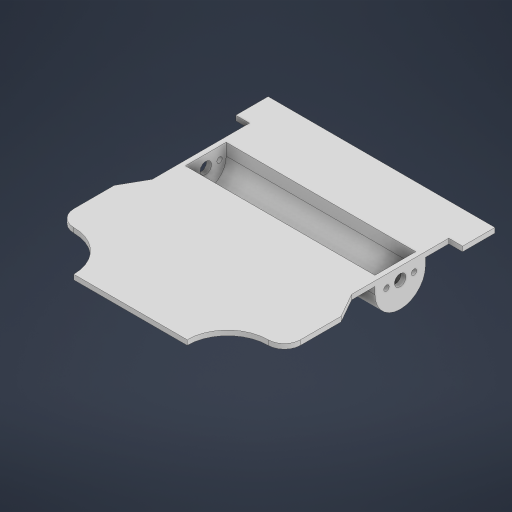
# Autodesk Inventor part: karoserie1
Saved by Autodesk Inventor 2023 (Build 270158000, 158)
## iProperties
Created: 2024-04-14
Part Number: karoserie1
Material: Generic
Document SubType Name: Modeling
Designer: Matooš
Density: 1 g/cm^3
Appearance: Default
Author: Matooš
Autodesk Inventor part; units mm, degrees
ref_plane "YZ Plane" through (0, 0, 0) normal (1, 0, 0) x (0, 1, 0)
ref_plane "XZ Plane" through (0, 0, 0) normal (0, 1, 0) x (-1, 0, 0)
ref_plane "XY Plane" through (0, 0, 0) normal (0, 0, 1) x (1, 0, 0)
sketch "Sketch1" plane through (0, 0, 0) normal (0, 1, 0) x (-1, 0, 0)
  line L0 (70, 45) -> (61.5, 30)
  line L1 (61.5, 30) -> (61.5, -30)
  line L2 (61.5, -30) -> (70, -30)
  line L3 (70, -30) -> (70, -50)
  line L4 (70, -50) -> (-70, -50)
  line L5 (-70, -50) -> (-70, -30)
  line L6 (-70, -30) -> (-61.5, -30)
  line L7 (-61.5, -30) -> (-61.5, 30)
  line L8 (-61.5, 30) -> (-70, 45)
  line L9 (70, 45) -> (70, 80)
  line L10 (-70, 45) -> (-70, 80)
  line L11 (35, 105) -> (-35, 105)
  line L12 (-98, 0) -> (98, 0) projected
  line L13 (0, -81) -> (0, 136) projected
  line L14 (70, 80) -> (35, 80)
  line L15 (35, 80) -> (35, 105)
  line L16 (-35, 105) -> (-35, 80)
  line L17 (-35, 80) -> (-70, 80)
  point P0 (0, 0)
  dimension "d0" = 60
  dimension "d1" = 60
  dimension "d2" = 123
  dimension "d3" = 140
  dimension "d4" = 20
  dimension "d5" = 140
  dimension "d8" = 35
  dimension "d15" = 30
  dimension "d45" = 15
  dimension "d46" = 15
  dimension "d47" = 35
  dimension "d48" = 70
  dimension "d49" = 155
  constraints: 32 end point, 9 perpendicular, 2 horizontal, 2 vertical, 1 collinear, 4 other
  measures "d0" distance of L0.end L1.end
  measures "d1" distance of L6.end L7.end
  measures "d2" distance between parallel lines of L7 L1
  measures "d3" distance of L3.end L4.end
  measures "d4" distance between parallel lines of L4 L2
  measures "d5" distance between parallel lines of L10 L9
  measures "d8" distance of L10.end L8.end
  measures "d15" distance between parallel lines of L12 L6
  measures "d45" vertical distance of L0.start L0.end
  measures "d46" vertical distance of L7.end L8.end
  measures "d47" distance of L0.start L9.end
  measures "d48" distance of L11.start L11.end
  measures "d49" distance between parallel lines of L4 L11
extrude "Extrusion1" add sketch "Sketch1" along normal blind 3
sketch "Sketch2" plane through (0, 0, 0) normal (0, -1, 0) x (1, 0, 0)
  line L0 (-98, 0) -> (98, 0) projected
  line L1 (0, 136) -> (0, -81) projected
  line L2 (61.5, 15.6) -> (58.5, 15.6)
  line L3 (58.5, 15.6) -> (58.5, -15.6)
  line L4 (58.5, -15.6) -> (61.5, -15.6)
  line L5 (61.5, -15.6) -> (61.5, 15.6)
  line L6 (61.5, 30) -> (61.5, -30) projected
  point P0 (0, 0)
  dimension "d18" = 3
  dimension "d19" = 31.2
  constraints: 8 end point, 2 parallel, 1 collinear, 1 horizontal, 1 perpendicular, 1 other
  measures "d18" distance between parallel lines of L5 L3
  measures "d19" distance of L4.end L2.start
extrude "Extrusion2" add sketch "Sketch2" along normal blind 20
sketch "Sketch3" plane through (61.5, 0, -30) normal (1, 0, 0) x (0, 0, -1)
  line L0 (-45.6, 0) -> (-45.6, -20) projected
  line L1 (-14.4, -20) -> (-45.6, -20) projected
  line L2 (-30, -24.6) -> (-30, 7.6) projected
  point P0 (-30, 0)
  point P1 (-38.5, -4.4)
  point P2 (-21.5, -4.4)
  dimension "d22" = 17
  dimension "d23" = 15.6
  constraints: 1 symmetric about line
  measures "d22" distance of point (-21.5, -4.4) point (-38.5, -4.4)
  measures "d23" distance from line of L1 point (-21.5, -4.4)
hole "Hole1" at (61.5, -4.4, 8.5) at (61.5, -4.4, -8.5) direction (-1, 0, 0) diameter 3.4 end through all clearance for "Countersunk Flat Head Screw ISO 2009/7046" size "M3" standard "ISO"
sketch "Sketch4" plane through (61.5, 0, -30) normal (1, 0, 0) x (0, 0, -1)
  line L0 (-30, -24.6) -> (-30, 7.6) projected
  circle A0 centre (-38.5, -4.4) radius 1.7 projected
  circle A1 centre (-21.5, -4.4) radius 1.7 projected
  line L1 (-38.5, -4.4) -> (-21.5, -4.4) construction
  point P0 (-30, 0)
  point P1 (-30, -4.4)
  constraints: 2 end point, 1 horizontal, 1 midpoint
hole "Hole2" at (61.5, -4.4, 0) direction (-1, 0, 0) diameter 7.1 end through all
fillet "Fillet1" radius 15.6 2 edges at (60, -20, -15.6) (60, -20, 15.6)
sketch "Sketch5" plane through (0, 0, 0) normal (1, 0, 0) x (0, 1, 0)
  line L0 (-24, 0) -> (4, 0) projected
  circle A0 centre (-4.4, 0) radius 3.55 projected
  arc A1 (-4.4, 12.6) -> (-4.4, -12.6) centre (-4.4, 0) ccw
  arc A2 (-4.4, 15.6) -> (-4.4, -15.6) centre (-4.4, 0) ccw
  line L1 (0, -15.6) -> (-4.4, -15.6) projected
  line L2 (-4.4, -15.6) -> (0, -15.6)
  line L3 (0, 30) -> (0, 15.6) projected
  line L4 (0, 15.6) -> (-4.4, 15.6) projected
  line L5 (-4.4, 15.6) -> (0, 15.6)
  line L6 (0, -15.6) -> (0, 15.6) projected
  line L7 (0, 15.6) -> (0, -15.6)
  line L8 (-4.4, 12.6) -> (0, 12.6)
  line L9 (-4.4, -12.6) -> (0, -12.6)
  point P0 (0, 0)
  point P1 (0, -12.6)
  point P2 (0, 12.6)
  dimension "d39" = 25.2
  dimension "d40" = 3
  constraints: 10 end point, 4 point on circle, 2 centre point, 2 coincident, 2 collinear, 2 perpendicular, 2 point on line, 2 tangent, 1 horizontal
  measures "d39" diameter of A1
  measures "d40" radial gap between concentric circles of A2 A1
extrude "Extrusion3" add sketch "Sketch5" along normal up to surface (58.5 mm away) contours A2 L4 L6 L8 A1 L0 | L0 A1 L9 L6 L1 A2
sketch "Sketch6" plane through (0, 0, 0) normal (1, 0, 0) x (0, 1, 0)
  line L0 (0, 42) -> (0, -42) projected
  line L1 (-5.88, 0) -> (4.48, 0) projected
  line L2 (3, 12.6) -> (0, 12.6)
  line L3 (0, 12.6) -> (0, -12.6)
  line L4 (0, -12.6) -> (3, -12.6)
  line L5 (3, -12.6) -> (3, 12.6)
  line L6 (0, -12.6) -> (-4.4, -12.6) projected
  line L7 (-4.4, 12.6) -> (0, 12.6) projected
  line L8 (3, -30) -> (3, 30) projected
  line L9 (0, -30) -> (0, 30) projected
  point P0 (0, 0)
  point P1 (0, 12.6)
  point P2 (0, -12.6)
  constraints: 8 end point, 4 collinear, 2 parallel, 1 horizontal, 1 perpendicular
extrude "Extrusion4" cut sketch "Sketch6" along normal mid plane 117
mirror "Mirror1" about plane through (0, 0, 0) normal (1, 0, 0) of "Hole1", "Hole2", "Extrusion2", "Fillet1", "Extrusion3"
fillet "Fillet2" radius 25 2 edges at (35, 1.5, 80) (-35, 1.5, 80)
fillet "Fillet3" radius 10 2 edges at (70, 1.5, 80) (-70, 1.5, 80)
body "Solid1"
